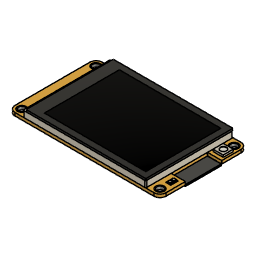
Console Enclosure Prototype v14 (Autodesk Fusion 360 archive; units mm, degrees)
design "ESP32-2432S024 Display"
Autodesk Fusion 360 part; units mm, degrees
note: some values were not read from the file. Chosen so that the rebuilt part matches the saved one: which bodies a step acts on. Set by a fixed rule: which sketch regions a step uses.
sketch "Sketch1" plane through (0, 0, 0) normal (0, 0, 1) x (1, 0, 0)
  line L0 (34, 18.25) -> (-34, 18.25)
  line L1 (-34, 18.25) -> (-34, -18.25)
  line L2 (-34, -18.25) -> (34, -18.25)
  line L3 (34, -18.25) -> (34, 18.25)
  line L4 (34, 18.25) -> (-34, -18.25) construction
  line L5 (-34, 18.25) -> (34, -18.25) construction
  line L6 (37.2, -18.45) -> (37.2, 18.45)
  line L7 (34.2, 21.45) -> (-34.2, 21.45)
  line L8 (-37.2, 18.45) -> (-37.2, -18.45)
  line L9 (-34.2, -21.45) -> (34.2, -21.45)
  circle A0 centre (-34, -18.25) radius 1.6
  circle A1 centre (-34, 18.25) radius 1.6
  circle A2 centre (34, 18.25) radius 1.6
  circle A3 centre (34, -18.25) radius 1.6
  arc A4 (37.2, 18.45) -> (34.2, 21.45) centre (34.2, 18.45) ccw
  arc A5 (34.2, -21.45) -> (37.2, -18.45) centre (34.2, -18.45) ccw
  arc A6 (-37.2, -18.45) -> (-34.2, -21.45) centre (-34.2, -18.45) ccw
  arc A7 (-34.2, 21.45) -> (-37.2, 18.45) centre (-34.2, 18.45) ccw
  line L10 (-30.2, 21.45) -> (30.2, 21.45)
  line L11 (30.2, 21.45) -> (30.2, -21.45)
  line L12 (30.2, -21.45) -> (-30.2, -21.45)
  line L13 (-30.2, -21.45) -> (-30.2, 21.45)
  circle A8 centre (34, 18.25) radius 2.1
  circle A9 centre (34, -18.25) radius 2.1
  circle A10 centre (-34, 18.25) radius 2.1
  circle A11 centre (-34, -18.25) radius 2.1
  line L14 (30.2, 8.95) -> (37.2, 8.95)
  line L15 (37.2, 8.95) -> (37.2, -8.95)
  line L16 (37.2, -8.95) -> (30.2, -8.95)
  line L17 (30.2, -8.95) -> (30.2, 8.95)
  line L18 (32.695, -10.45) -> (35.1716, -10.45)
  line L19 (35.1716, -10.45) -> (35.1716, -14.15)
  line L20 (35.1716, -14.15) -> (32.695, -14.15)
  line L21 (32.695, -14.15) -> (32.695, -10.45)
  line L22 (33.2332, -10.55) -> (34.6279, -10.55)
  line L23 (34.6279, -10.55) -> (34.6279, -12.05)
  line L24 (34.6279, -12.05) -> (33.2332, -12.05)
  line L25 (33.2332, -12.05) -> (33.2332, -10.55)
  line L26 (33.2332, -12.55) -> (34.6279, -12.55)
  line L27 (34.6279, -12.55) -> (34.6279, -14.05)
  line L28 (34.6279, -14.05) -> (33.2332, -14.05)
  line L29 (33.2332, -14.05) -> (33.2332, -12.55)
  line L30 (32.695, -12.3) -> (35.1716, -12.3)
  dimension "d1" = 68
  dimension "d2" = 36.5
  dimension "d4" = 3.2
  dimension "d5" = 3.2
  dimension "d6" = 3.2
  dimension "d7" = 3.2
  dimension "d8" = 3
  dimension "d9" = 7
  dimension "d10" = 7
  dimension "d11" = 0.5
  dimension "d12" = 0.5
  dimension "d13" = 0.5
  dimension "d14" = 0.5
  dimension "d35" = 12.5
  dimension "d36" = 12.5
  dimension "d41" = 4.1
  dimension "d42" = 1.5
  dimension "d43" = 0.1
  dimension "d44" = 0.1
  dimension "d45" = 0.25
  dimension "d46" = 0.25
  constraint horizontal L0
  constraint perpendicular L0 L1
  constraint parallel L0 L2
  constraint parallel L1 L3
  constraint coincident L4 origin
  constraint coincident L5 origin
  constraint coincident L1.end L2.start
  constraint coincident L0.end L1.start
  constraint coincident L0.start L3.end
  constraint coincident L2.end L3.start
  constraint tangent L6 A4
  constraint tangent L7 A4
  constraint tangent L6 A5
  constraint tangent L9 A5
  constraint equal A4 A5
  constraint tangent L8 A6
  constraint tangent L9 A6
  constraint equal A4 A6
  constraint tangent L7 A7
  constraint tangent L8 A7
  constraint equal A4 A7
  constraint horizontal L10
  constraint vertical L11
  constraint horizontal L12
  constraint vertical L13
  constraint coincident L9 L11.end
  constraint coincident L7 L10.start
  constraint horizontal L14
  constraint vertical L15
  constraint horizontal L16
  constraint vertical L17
  constraint coincident L6 L15.end
  constraint coincident L11 L14.start
  constraint horizontal L18
  constraint vertical L19
  constraint horizontal L20
  constraint vertical L21
  constraint horizontal L22
  constraint vertical L23
  constraint horizontal L24
  constraint vertical L25
  constraint horizontal L26
  constraint vertical L27
  constraint horizontal L28
  constraint vertical L29
  constraint midpoint L21 L30.start
  constraint midpoint L19 L30.end
  measures "d1" distance of L1.end L2.end
  measures "d2" distance of L0.end L1.end
  measures "d4" diameter of A0
  measures "d5" diameter of A1
  measures "d6" diameter of A2
  measures "d7" diameter of A3
  measures "d8" radius of A4
  measures "d9" distance of L6 L11
  measures "d10" distance of L8 L13
  measures "d35" distance of L7 L14
  measures "d36" distance of L9 L16
  measures "d41" distance of L2.end L20
  measures "d42" distance of L16 L18
  measures "d43" distance of L18 L22
  measures "d44" distance of L20 L28
  measures "d45" distance of L26 L30
  measures "d46" distance of L24 L30
extrude "Extrude1" add sketch "Sketch1" along normal blind 1.5 contours L0 L1 A1 A10 | L0 L1 L2 L7 L8 L9 A6 A7 L13 A10 A11 | L0 L1 A1 A10 | L0 L1 L2 L13 A10 A11 | L0 L7 L10 L11 L13 | L0 L2 L11 L13 L17 | L0 L3 L6 L7 A4 L11 A8 L14 | L0 L3 L11 A8 L14 | L2 L9 L11 L12 L13 | L1 L2 A0 A11 | L1 L2 A0 A11 | L0 L3 A2 A8 | L0 L3 A2 A8 | L3 L11 L14 L16 L17 | L2 L3 L11 A9 L16 L18 L20 L21 | L2 L3 L6 L9 A5 L11 A9 L16 L18 L19 L20 | L3 L6 L14 L15 L16 | L2 L3 A3 A9 | L2 L3 A3 A9 | L3 L18 L19 L22 L23 L24 L30 | L3 L18 L21 L22 L24 L25 L30 | L3 L20 L21 L26 L28 L29 L30 | L3 L19 L20 L26 L27 L28 L30 | L3 L22 L23 L24 | L3 L22 L24 L25 | L3 L26 L28 L29 | L3 L26 L27 L28 makes body 1
split "Split1" by curves path "Sketch1" along A11 A8 A9 A10 bodies 1 makes body 2 at (-10.7027, -5.7796, 0) makes body 3 at (32.402, -18.3298, 0.5) makes body 4 at (34.934, 19.5491, 1) makes body 5 at (-34, 19.85, 1)
sketch "Sketch2" plane through (0, 0, 1.5) normal (0, 0, 1) x (-1, 0, 0)
  circle A0 centre (34, -18.25) radius 2.1
  circle A1 centre (-34, -18.25) radius 2.1
  circle A2 centre (34, 18.25) radius 2.1
  circle A3 centre (-34, 18.25) radius 2.1
  arc A4 (-34.2, 21.45) -> (-37.2, 18.45) centre (-34.2, 18.45) ccw
  line L0 (-37.2, 18.45) -> (-37.2, -18.45)
  arc A5 (-37.2, -18.45) -> (-34.2, -21.45) centre (-34.2, -18.45) ccw
  line L1 (-34.2, -21.45) -> (34.2, -21.45)
  arc A6 (34.2, -21.45) -> (37.2, -18.45) centre (34.2, -18.45) ccw
  line L2 (37.2, -18.45) -> (37.2, 18.45)
  arc A7 (37.2, 18.45) -> (34.2, 21.45) centre (34.2, 18.45) ccw
  line L3 (34.2, 21.45) -> (-34.2, 21.45)
sketch "Sketch1 (2)" plane through (0, 0, 1.5) normal (0, 0, 1) x (-1, 0, 0) in component "Screen"
  line L0 (-34.2, -21.45) -> (34.2, -21.45)
  line L1 (-30.2, 21.45) -> (30.2, 21.45)
  line L2 (34.2, 21.45) -> (-34.2, 21.45)
  arc A0 (37.2, 18.45) -> (34.2, 21.45) centre (34.2, 18.45) ccw
  line L3 (37.2, -18.45) -> (37.2, 18.45)
  arc A1 (34.2, -21.45) -> (37.2, -18.45) centre (34.2, -18.45) ccw
  arc A2 (-37.2, -18.45) -> (-34.2, -21.45) centre (-34.2, -18.45) ccw
  line L4 (-37.2, 18.45) -> (-37.2, -18.45)
  arc A3 (-34.2, 21.45) -> (-37.2, 18.45) centre (-34.2, 18.45) ccw
  line L5 (30.2, -21.45) -> (-30.2, -21.45)
  line L6 (-30.2, -21.45) -> (-30.2, 21.45)
  line L7 (-30.2, 21.45) -> (30.2, 21.45)
  line L8 (30.2, 21.45) -> (30.2, -21.45)
  line L9 (28.7, -21.45) -> (28.7, 21.45)
  dimension "d17" = 7
  dimension "d18" = 7
  dimension "d19" = 1.5
  constraint horizontal L5
  constraint vertical L6
  constraint horizontal L7
  constraint vertical L8
  constraint coincident L1 L6.end
  constraint coincident L0 L5.start
  constraint coincident L5 L9.start
  constraint coincident L1 L9.end
  constraint perpendicular L1 L9
  measures "d17" distance of L4 L6
  measures "d18" distance of L3 L8
  measures "d19" distance of L8 L9
extrude "Extrude1'" add sketch "Sketch1 (2)" along normal blind 3 separate body contours L0 L1 L2 L5 L6 L7 L9 | L0 L1 L2 L5 L7 L8 L9 makes body 6 in component "Screen"
extrude "Extrude2" add sketch "Sketch1 (2)" along normal blind 1 from surface at 3 separate body contours L0 L1 L2 L5 L6 L7 L9 makes body 7 in component "Screen"
sketch "Sketch1 (3)" plane through (0, 0, 1.5) normal (0, 0, 1) x (-1, 0, 0) in component "RGB-LED"
  line L0 (-31.2, -15.65) -> (-36.2, -15.65)
  line L1 (-36.2, -15.65) -> (-36.2, -10.65)
  line L2 (-36.2, -10.65) -> (-31.2, -10.65)
  line L3 (-31.2, -10.65) -> (-31.2, -15.65)
  circle A0 centre (-34, -18.25) radius 2.1
  line L4 (-37.2, 18.45) -> (-37.2, -18.45)
  circle A1 centre (-33.7, -13.3) radius 1.5
  dimension "d25" = 5
  dimension "d26" = 5
  dimension "d27" = 2.6
  dimension "d28" = 1
  dimension "d29" = 3
  constraint horizontal L0
  constraint vertical L1
  constraint horizontal L2
  constraint vertical L3
  measures "d25" distance of L0.start L0.end
  measures "d26" distance of L0.start L2.end
  measures "d27" distance of L0 A0.centre
  measures "d28" distance of L1 L4
  measures "d29" diameter of A1
extrude "Extrude1''" add sketch "Sketch1 (3)" along normal blind 1 separate body contours L0 L1 L2 L3 | A1 makes body 8 in component "RGB-LED"
extrude "Extrude2'" cut sketch "Sketch1 (3)" against normal blind 0.2 from surface at 1 contours A1 bodies 8 in component "RGB-LED"
extrude "Extrude2''" cut sketch "Sketch1" along normal blind 3 contours L3 L11 L14 L16 L17 | L3 L6 L14 L15 L16 bodies 2
fillet "Fillet1" radius 0.1 4 edges at (37.2, 8.95, 0.75) (37.2, -8.95, 0.75) (30.2, -8.95, 0.75) (30.2, 8.95, 0.75) on bodies 2
split "Split4" by curves path "Sketch1" along L21 L18 L19 L20 bodies 2 makes body 9 at (-11.4433, 2.95, 0)
split "Split5" by curves path "Sketch1" along L29 L26 L27 L28 bodies 2 makes body 10 at (34.1648, -11.15, 0)
split "Split6" by curves path "Sketch1" along L25 L22 L23 L24 bodies 10 makes body 11 at (35.1716, -11.6833, 0.5)
sketch "Sketch1 (4)" plane through (0, 0, 1.5) normal (0, 0, 1) x (-1, 0, 0) in component "Resistor"
  line L0 (-33.2332, 12.05) -> (-33.2332, 10.55)
  line L1 (-33.2332, 10.55) -> (-34.6279, 10.55)
  line L2 (-34.6279, 10.55) -> (-34.6279, 12.05)
  line L3 (-34.6279, 12.05) -> (-33.2332, 12.05)
  line L4 (-33.2332, 14.05) -> (-33.2332, 12.55)
  line L5 (-33.2332, 12.55) -> (-34.6279, 12.55)
  line L6 (-34.6279, 12.55) -> (-34.6279, 14.05)
  line L7 (-34.6279, 14.05) -> (-33.2332, 14.05)
  line L8 (-32.695, 10.45) -> (-32.695, 14.15)
  line L9 (-32.695, 14.15) -> (-35.1716, 14.15)
  line L10 (-35.1716, 14.15) -> (-35.1716, 10.45)
  line L11 (-35.1716, 10.45) -> (-32.695, 10.45)
  line L12 (-33.2332, 10.75) -> (-34.6279, 10.75)
  line L13 (-34.6279, 10.75) -> (-34.6279, 13.85)
  line L14 (-34.6279, 13.85) -> (-33.2332, 13.85)
  line L15 (-33.2332, 13.85) -> (-33.2332, 10.75)
  line L16 (-34.6279, 14.05) -> (-33.2332, 14.05)
  line L17 (-33.2332, 10.55) -> (-34.6279, 10.55)
  dimension "d47" = 0.2
  dimension "d48" = 0.2
  constraint horizontal L12
  constraint vertical L13
  constraint horizontal L14
  constraint vertical L15
  constraint coincident L6 L13.end
  constraint coincident L0 L12.start
  measures "d47" distance of L14 L16
  measures "d48" distance of L12 L17
extrude "Extrude1'''" add sketch "Sketch1 (4)" along normal blind 0.5 separate body contours L0 L2 L3 L12 L13 L15 | L3 L5 L13 L15 | L4 L5 L6 L13 L14 L15 makes body 12 in component "Resistor"
split "Split1'" by curves path "Sketch1 (4)" along L7 L4 L5 L6 bodies 12 makes body 13 at (34.163, -11.6167, 1.5) in component "Resistor"
split "Split2" by curves path "Sketch1 (4)" along L1 L2 L3 L0 bodies 13 makes body 14 at (33.6981, -12.55, 1.6667) in component "Resistor"
fillet "Fillet1'" radius 0.05 8 edges at (33.9306, -13.85, 2) (33.2332, -13.2, 2) (34.6279, -13.2, 2) (33.2332, -11.4, 2) (33.9306, -10.75, 2) (34.6279, -11.4, 2) (33.2332, -12.3, 2) (34.6279, -12.3, 2) on bodies 12 13 14 in component "Resistor"
sketch "Sketch1 (5)" plane through (0, 0, 0) normal (0, 0, -1) x (1, 0, 0) in component "ESP32"
  line L0 (32.695, 10.45) -> (32.695, 14.15)
  line L1 (32.695, 14.15) -> (35.1716, 14.15)
  line L2 (35.1716, 14.15) -> (35.1716, 10.45)
  line L3 (35.1716, 10.45) -> (32.695, 10.45)
  arc A0 (37.1, 8.95) -> (37.2, 9.05) centre (37.1, 9.05) ccw
  line L4 (37.2, 9.05) -> (37.2, 18.45)
  arc A1 (37.2, 18.45) -> (34.2, 21.45) centre (34.2, 18.45) ccw
  line L5 (34.2, 21.45) -> (-34.2, 21.45)
  arc A2 (-34.2, 21.45) -> (-37.2, 18.45) centre (-34.2, 18.45) ccw
  line L6 (-37.2, 18.45) -> (-37.2, -18.45)
  arc A3 (-37.2, -18.45) -> (-34.2, -21.45) centre (-34.2, -18.45) ccw
  line L7 (-34.2, -21.45) -> (34.2, -21.45)
  arc A4 (34.2, -21.45) -> (37.2, -18.45) centre (34.2, -18.45) ccw
  line L8 (37.2, -18.45) -> (37.2, -9.05)
  arc A5 (37.2, -9.05) -> (37.1, -8.95) centre (37.1, -9.05) ccw
  line L9 (37.1, -8.95) -> (30.3, -8.95)
  arc A6 (30.2, -8.85) -> (30.3, -8.95) centre (30.3, -8.85) ccw
  line L10 (30.2, -8.85) -> (30.2, 8.85)
  arc A7 (30.3, 8.95) -> (30.2, 8.85) centre (30.3, 8.85) ccw
  line L11 (30.3, 8.95) -> (37.1, 8.95)
  circle A8 centre (-34, -18.25) radius 2.1
  circle A9 centre (34, -18.25) radius 2.1
  circle A10 centre (-34, 18.25) radius 2.1
  circle A11 centre (34, 18.25) radius 2.1
  line L12 (30.2, -8.85) -> (30.2, 8.85)
  line L13 (30.3, 8.95) -> (37.1, 8.95)
  line L14 (37.1, -8.95) -> (30.3, -8.95)
  line L15 (30.3, 8.95) -> (12.8, 8.95)
  line L16 (12.8, 8.95) -> (12.8, -8.95)
  line L17 (12.8, -8.95) -> (30.3, -8.95)
  line L18 (30.3, -8.95) -> (30.3, 8.95)
  line L19 (13.3, 8.45) -> (13.3, -8.45)
  line L20 (13.3, -8.45) -> (29.8, -8.45)
  line L21 (29.8, -8.45) -> (29.8, 8.45)
  line L22 (29.8, 8.45) -> (13.3, 8.45)
  line L23 (37.1, 8.95) -> (37.1, -8.95)
  line L24 (30.3, 8.85) -> (37, 8.85)
  line L25 (37, 8.85) -> (37, -8.85)
  line L26 (37, -8.85) -> (30.3, -8.85)
  dimension "d53" = 17.5
  dimension "d55" = 0.1
  constraint horizontal L15
  constraint vertical L16
  constraint horizontal L17
  constraint vertical L18
  constraint coincident A7.start L11.start
  constraint coincident A5.end L9.start
  constraint coincident L9.end A6.end
  constraint coincident A0.start L11.end
  measures "d53" distance of A7.start L15.end
extrude "Extrude1''''" add sketch "Sketch1 (5)" along normal blind 0.8 separate body contours L9 L11 L13 L14 L18 L23 L24 L25 L26 | A6 L10 A7 L12 L18 | A6 L10 A7 L12 L15 L16 L17 | L18 L24 L25 L26 | L19 L20 L21 L22 makes body 15 in component "ESP32"
extrude "Extrude2'''" add sketch "Sketch1 (5)" along normal blind 2 from surface at 0.8 separate body contours L19 L20 L21 L22 makes body 16 in component "ESP32"
fillet "Fillet1''" radius 0.1 16 edges at (24.95, 8.95, -0.8) (12.8, 0, -0.8) (37.1, 0, -0.8) (24.95, -8.95, -0.8) (37.1, 0, 0) (24.95, -8.95, 0) (37.1, -8.95, -0.4) (37.1, 8.95, -0.4) (12.8, 8.95, -0.4) (24.95, 8.95, 0) (12.8, 0, 0) (12.8, -8.95, -0.4) (21.55, 8.45, -2.8) (13.3, 0, -2.8) (21.55, -8.45, -2.8) (29.8, 0, -2.8) on bodies 15 16 in component "ESP32"
fillet "Fillet2" radius 0.1 8 edges at (13.3, -8.45, -1.75) (13.3293, -8.4207, -2.7707) (13.3, 8.45, -1.75) (13.3293, 8.4207, -2.7707) (29.8, -8.45, -1.75) (29.7707, -8.4207, -2.7707) (29.8, 8.45, -1.75) (29.7707, 8.4207, -2.7707) on bodies 16 in component "ESP32"
fillet "Fillet1'''" radius 0.5 4 edges at (-30.2, -21.45, 3) (-30.2, 21.45, 3) (30.2, 21.45, 3) (30.2, -21.45, 3) on bodies 6 7 in component "Screen"
fillet "Fillet1'''" radius 0.25 4 edges at (30.2, -21.45, 5) (-28.7, -21.45, 5) (-28.7, 21.45, 5) (30.2, 21.45, 5) on bodies 6 7 in component "Screen"
sketch "Sketch2 (2)" plane through (0, 0, 5.5) normal (0, 0, 1) x (-1, 0, 0) in component "Screen"
  arc A0 (-30.2, -21.2) -> (-29.95, -21.45) centre (-29.95, -21.2) ccw
  line L0 (-29.95, -21.45) -> (28.45, -21.45)
  arc A1 (28.45, -21.45) -> (28.7, -21.2) centre (28.45, -21.2) ccw
  line L1 (28.7, -21.2) -> (28.7, 21.2)
  arc A2 (28.7, 21.2) -> (28.45, 21.45) centre (28.45, 21.2) ccw
  line L2 (28.45, 21.45) -> (-29.95, 21.45)
  arc A3 (-29.95, 21.45) -> (-30.2, 21.2) centre (-29.95, 21.2) ccw
  line L3 (-30.2, 21.2) -> (-30.2, -21.2)
  line L4 (22.7, -18.45) -> (-27.2, -18.45)
  line L5 (-27.2, -18.45) -> (-27.2, 18.45)
  line L6 (-27.2, 18.45) -> (22.7, 18.45)
  line L7 (22.7, 18.45) -> (22.7, -18.45)
  line L8 (-30.2, -21.45) -> (-30.2, 21.45)
  line L9 (-30.2, 21.45) -> (30.2, 21.45)
  line L10 (30.2, -21.45) -> (-30.2, -21.45)
  line L11 (28.7, -21.45) -> (28.7, 21.45)
  dimension "d69" = 3
  dimension "d70" = 3
  dimension "d71" = 3
  dimension "d72" = 6
  constraint horizontal L4
  constraint vertical L5
  constraint horizontal L6
  constraint vertical L7
  measures "d69" distance of L5 L8
  measures "d70" distance of L6 L9
  measures "d71" distance of L4 L10
  measures "d72" distance of L7 L11
split "Split1''" by curves path "Sketch2 (2)" along L5 L6 L7 L4 bodies 7 makes body 17 at (-26.7, -6.15, 4.5) in component "Screen"
sketch "Sketch3" plane through (0, 0, 0) normal (0, 0, -1) x (1, 0, 0)
  line L0 (32.695, 10.45) -> (32.695, 14.15)
  line L1 (32.695, 14.15) -> (35.1716, 14.15)
  line L2 (35.1716, 14.15) -> (35.1716, 10.45)
  line L3 (35.1716, 10.45) -> (32.695, 10.45)
  arc A0 (37.1, 8.95) -> (37.2, 9.05) centre (37.1, 9.05) ccw
  line L4 (37.2, 9.05) -> (37.2, 18.45)
  arc A1 (37.2, 18.45) -> (34.2, 21.45) centre (34.2, 18.45) ccw
  line L5 (34.2, 21.45) -> (-34.2, 21.45)
  arc A2 (-34.2, 21.45) -> (-37.2, 18.45) centre (-34.2, 18.45) ccw
  line L6 (-37.2, 18.45) -> (-37.2, -18.45)
  arc A3 (-37.2, -18.45) -> (-34.2, -21.45) centre (-34.2, -18.45) ccw
  line L7 (-34.2, -21.45) -> (34.2, -21.45)
  arc A4 (34.2, -21.45) -> (37.2, -18.45) centre (34.2, -18.45) ccw
  line L8 (37.2, -18.45) -> (37.2, -9.05)
  arc A5 (37.2, -9.05) -> (37.1, -8.95) centre (37.1, -9.05) ccw
  line L9 (37.1, -8.95) -> (30.3, -8.95)
  arc A6 (30.2, -8.85) -> (30.3, -8.95) centre (30.3, -8.85) ccw
  line L10 (30.2, -8.85) -> (30.2, 8.85)
  arc A7 (30.3, 8.95) -> (30.2, 8.85) centre (30.3, 8.85) ccw
  line L11 (30.3, 8.95) -> (37.1, 8.95)
  circle A8 centre (-34, -18.25) radius 2.1
  circle A9 centre (34, -18.25) radius 2.1
  circle A10 centre (-34, 18.25) radius 2.1
  circle A11 centre (34, 18.25) radius 2.1
  line L12 (-37.2, -6.95) -> (-29.7, -6.95)
  line L13 (-29.7, -6.95) -> (-29.7, 2.05)
  line L14 (-29.7, 2.05) -> (-37.2, 2.05)
  line L15 (-37.2, 2.05) -> (-37.2, -6.95)
  point P0 (-30.2, -21.45)
  dimension "d73" = 9
  dimension "d74" = 7.5
  dimension "d75" = 14.5
  constraint horizontal L12
  constraint vertical L13
  constraint horizontal L14
  constraint vertical L15
  constraint coincident L6 L12.start
  measures "d73" distance of L12.end L13.end
  measures "d74" distance of L12.start L12.end
  measures "d75" distance of L12 P0
extrude "Extrude3" add sketch "Sketch3" along normal blind 3 separate body contours L6 L12 L13 L14 L15 makes body 18
fillet "Fillet2'" radius 1 4 edges at (-33.45, -2.05, -3) (-33.45, -2.05, 0) (-33.45, 6.95, -3) (-33.45, 6.95, 0) on bodies 18
sketch "Sketch4" plane through (-37.2, 0, 0) normal (-1, 0, 0) x (0, -1, 0)
  arc A0 (-5.95, 0) -> (-6.95, -1) centre (-5.95, -1) ccw
  line L0 (-6.95, -1) -> (-6.95, -2)
  arc A1 (-6.95, -2) -> (-5.95, -3) centre (-5.95, -2) ccw
  line L1 (-5.95, -3) -> (1.05, -3)
  arc A2 (1.05, -3) -> (2.05, -2) centre (1.05, -2) ccw
  line L2 (2.05, -2) -> (2.05, -1)
  arc A3 (2.05, -1) -> (1.05, 0) centre (1.05, -1) ccw
  line L3 (1.05, 0) -> (-5.95, 0)
  line L4 (1.75, -2) -> (1.75, -1)
  arc A4 (1.75, -1) -> (1.05, -0.3) centre (1.05, -1) ccw
  line L5 (1.05, -0.3) -> (-5.95, -0.3)
  arc A5 (-5.95, -0.3) -> (-6.65, -1) centre (-5.95, -1) ccw
  line L6 (-6.65, -1) -> (-6.65, -2)
  arc A6 (-6.65, -2) -> (-5.95, -2.7) centre (-5.95, -2) ccw
  line L7 (-5.95, -2.7) -> (1.05, -2.7)
  arc A7 (1.05, -2.7) -> (1.75, -2) centre (1.05, -2) ccw
  dimension "d80" = -0.3
extrude "Extrude4" cut sketch "Sketch4" against normal blind 7 contours L4 A4 L5 A5 L6 A6 L7 A7 bodies 18
sketch "Sketch5" plane through (-30.2, 0, 0) normal (-1, 0, 0) x (0, -1, 0)
  arc A0 (1.05, -2.7) -> (1.75, -2) centre (1.05, -2) ccw
  line L0 (1.75, -2) -> (1.75, -1)
  arc A1 (1.75, -1) -> (1.05, -0.3) centre (1.05, -1) ccw
  line L1 (1.05, -0.3) -> (-5.95, -0.3)
  arc A2 (-5.95, -0.3) -> (-6.65, -1) centre (-5.95, -1) ccw
  line L2 (-6.65, -1) -> (-6.65, -2)
  arc A3 (-6.65, -2) -> (-5.95, -2.7) centre (-5.95, -2) ccw
  line L3 (-5.95, -2.7) -> (1.05, -2.7)
  line L4 (1.05, -2) -> (-5.95, -2)
  line L5 (-5.95, -2) -> (-5.95, -1)
  line L6 (-5.95, -1) -> (1.05, -1)
  line L7 (1.05, -1) -> (1.05, -2)
  constraint horizontal L4
  constraint vertical L5
  constraint horizontal L6
  constraint vertical L7
  constraint coincident A2.centre L5.end
  constraint coincident A0.centre L4.start
extrude "Extrude5" add sketch "Sketch5" along normal up to surface (7 mm away) contours L4 L5 L6 L7 bodies 18
fillet "Fillet3" radius 0.5 4 edges at (-33.7, -1.05, -2) (-33.7, -1.05, -1) (-33.7, 5.95, -2) (-33.7, 5.95, -1) on bodies 18
component "Screen" placed x (1, 0, 0) y (0, 1, 0) z (0, 0, 1) at (0, 0, 0)
component "RGB-LED" placed x (1, 0, 0) y (0, 1, 0) z (0, 0, 1) at (0, 0, 0)
component "Resistor" placed x (1, 0, 0) y (0, 1, 0) z (0, 0, 1) at (0, 0, 0)
component "ESP32" placed x (1, 0, 0) y (0, 1, 0) z (0, 0, 1) at (0, 0, 0)
named bodies: "Rim1", "Resistorplate2", "Rim2", "Rim3", "Rim4", "Display-Lower", "Display-Screen", "Plate (1)", "Resistorplate", "Resistorplatform", "Display-Frame"
